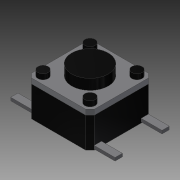
# Autodesk Inventor part: PZ_PushButton
Saved by Autodesk Inventor 2015 (Build 190159000, 159)
## iProperties
Created: 2015-10-19
Part Number: PZ_PushButton
Material: Genérico
Document SubType Name: Modeling
Designer: X1
Density: 1 g/cm^3
Appearance: Valor por defecto
Author: X1
Autodesk Inventor part; units mm, degrees
ref_plane "YZ Plane" through (0, 0, 0) normal (1, 0, 0) x (0, 1, 0)
ref_plane "XZ Plane" through (0, 0, 0) normal (0, 1, 0) x (-1, 0, 0)
sketch "Boceto1" plane through (0, 0, 0) normal (0, 0, 1) x (1, 0, 0)
  line L0 (-7.8, 0) -> (4.8, 0) projected
  line L1 (0, -4.2) -> (0, 4.2) projected
  line L2 (-2.6, 3) -> (2.6, 3)
  line L3 (3, 2.6) -> (3, -2.6)
  line L4 (2.6, -3) -> (-2.6, -3)
  line L5 (-3, -2.6) -> (-3, 2.6)
  circle A0 centre (-2.25, 2.25) radius 0.5
  circle A1 centre (-2.25, -2.25) radius 0.5
  circle A2 centre (2.25, 2.25) radius 0.5
  circle A3 centre (2.25, -2.25) radius 0.5
  circle A4 centre (0, 0) radius 1.75
  line L6 (-2.6, 3) -> (-3, 2.6)
  line L7 (2.6, 3) -> (3, 2.6)
  line L8 (3, -2.6) -> (2.6, -3)
  line L9 (-3, -2.6) -> (-2.6, -3)
  point P0 (-3, 3)
  point P1 (3, -3)
  point P2 (3, 3)
  point P3 (-3, -3)
  dimension "d0" = 6
  dimension "d1" = 6
  dimension "d2" = 4.5
  dimension "d4" = 4.5
  dimension "d5" = 1
  dimension "d6" = 3.5
  dimension "d7" = 0.4
  dimension "d8" = 0.4
  dimension "d9" = 0.4
  dimension "d10" = 0.4
  dimension "d11" = 0.4
  dimension "d12" = 0.4
  dimension "d13" = 0.4
  dimension "d14" = 0.4
  constraints: 16 end point, 8 point on line, 5 centre point, 2 parallel, 1 coincident, 1 horizontal, 1 perpendicular, 5 other
  measures "d0" distance of point (3, -3) point (-3, -3)
  measures "d1" distance of point (3, 3) point (3, -3)
  measures "d2" distance of A0.centre A1.centre
  measures "d4" distance of A2.centre A0.centre
  measures "d5" diameter of A0
  measures "d6" diameter of A4
  measures "d7" distance of L2.start point (-3, 3)
  measures "d8" distance of L5.end point (-3, 3)
  measures "d9" distance of L2.end point (3, 3)
  measures "d10" distance of L3.start point (3, 3)
  measures "d11" distance of L3.end point (3, -3)
  measures "d12" distance of L4.start point (3, -3)
  measures "d13" distance of L5.start point (-3, -3)
  measures "d14" distance of L4.end point (-3, -3)
extrude "Extrusión1" add sketch "Boceto1" against normal blind 3.4 contours L5 L6 L2 L1 A4 L0 | L0 A4 L1 L4 L9 L5 | A4 L1 L0 | L0 L1 A4 | L1 A4 L0 | L0 A4 L1 | L1 L2 L7 L3 L0 A4 | A4 L0 L3 L8 L4 L1 | A0 | A1 | A2 | A3
extrude "Extrusión2" add sketch "Boceto1" along normal blind 0.5 contours A0 | A1 | A2 | A3
extrude "Extrusión3" add sketch "Boceto1" along normal blind 1 contours A4 L1 L0 | L0 L1 A4 | L1 A4 L0 | L0 A4 L1
ref_plane "Plano de trabajo1" through (0, 0, -3) normal (0, 0, 1) x (1, 0, 0)
sketch "Boceto2" plane through (0, 0, -3) normal (0, 0, 1) x (1, 0, 0)
  line L0 (-3, 2.6) -> (-2.6, 3) projected
  line L1 (-2.6, 3) -> (2.6, 3) projected
  line L2 (2.6, 3) -> (3, 2.6) projected
  line L3 (3, 2.6) -> (3, -2.6) projected
  line L4 (3, -2.6) -> (2.6, -3) projected
  line L5 (2.6, -3) -> (-2.6, -3) projected
  line L6 (-2.6, -3) -> (-3, -2.6) projected
  line L7 (-3, -2.6) -> (-3, 2.6) projected
  line L8 (-3, 2.6) -> (-5, 2.6)
  line L9 (-5, 2.6) -> (-5, 1.9)
  line L10 (-5, 1.9) -> (-3, 1.9)
  line L11 (-3, 1.9) -> (-3, 2.6)
  line L12 (-5, 2.25) -> (-3, 2.25)
  line L13 (-7.8, 0) -> (4.8, 0) projected
  line L14 (0, -4.2) -> (0, 4.2) projected
  line L15 (-3, -1.9) -> (-5, -1.9)
  line L16 (-5, -1.9) -> (-5, -2.6)
  line L17 (-5, -2.6) -> (-3, -2.6)
  line L18 (-3, -2.6) -> (-3, -1.9)
  line L19 (5, 2.6) -> (3, 2.6)
  line L20 (3, 2.6) -> (3, 1.9)
  line L21 (3, 1.9) -> (5, 1.9)
  line L22 (5, 1.9) -> (5, 2.6)
  line L23 (5, -1.9) -> (3, -1.9)
  line L24 (3, -1.9) -> (3, -2.6)
  line L25 (3, -2.6) -> (5, -2.6)
  line L26 (5, -2.6) -> (5, -1.9)
  point P0 (0, 0)
  point P1 (-5, -2.25)
  point P2 (-3, -2.25)
  point P3 (3, 2.25)
  point P4 (5, 2.25)
  point P5 (3, -2.25)
  point P6 (5, -2.25)
  dimension "d22" = 2
  dimension "d23" = 0.7
  dimension "d24" = 0.75
  dimension "d27" = 4.5
  dimension "d30" = 8
  constraints: 34 end point, 2 horizontal, 2 midpoint, 2 parallel, 1 perpendicular, 1 point on line, 1 vertical, 30 other
  measures "d22" distance of L10.end L9.end
  measures "d23" distance of L9.end L8.end
  measures "d24" distance between parallel lines of L1 L12
  measures "d27" distance of L9.end L17.start
  measures "d30" distance of L9.end L21.start
extrude "Extrusión4" add sketch "Boceto2" against normal blind 0.3 contours L7 L12 L9 L8 | L7 L10 L9 L12 | L19 L22 L21 L3 | L7 L17 L16 L15 | L23 L26 L25 L3
sketch "Boceto3" plane through (-2.6, 3, 0) normal (0, 1, 0) x (1, 0, 0)
  line L0 (5.2, 0) -> (0, 0) projected
  line L1 (5.2, 0) -> (5.2, 3.4) projected
  line L2 (0, 3.4) -> (5.2, 3.4) projected
  line L3 (0, 0) -> (0, 3.4) projected
  line L4 (5.2, 0.5) -> (0, 0.5)
  line L5 (0, 0) -> (0, 3.4) projected
  point P0 (2.6, 0)
  dimension "d35" = 0.5
  constraints: 2 end point, 2 point on line, 1 perpendicular
  measures "d35" distance between parallel lines of L0 L4
extrude "Extrusión5" add sketch "Boceto3" along normal blind 0.0001 contours L0 L3 L4 L1
mirror "Simetría1" about plane through (0, 0, 0) normal (0, 1, 0) of "Extrusión5"
sketch "Boceto4" plane through (3, -2.6, 0) normal (1, 0, 0) x (0, 0, -1)
  line L0 (3.3, 5.2) -> (3.3, 4.5) projected
  line L1 (3.3, 4.5) -> (3, 4.5) projected
  line L2 (3, 4.5) -> (3, 5.2) projected
  line L3 (0, 5.2) -> (3, 5.2) projected
  line L4 (0, 0) -> (0, 5.2) projected
  line L5 (0, 0) -> (3, 0) projected
  line L6 (3, 0) -> (3, 0.7) projected
  line L7 (3, 0.7) -> (3.3, 0.7) projected
  line L8 (3.3, 0.7) -> (3.3, 0) projected
  line L9 (3.3, 0) -> (3.4, 0) projected
  line L10 (3.4, 5.2) -> (3.4, 0) projected
  line L11 (3.3, 5.2) -> (3.4, 5.2) projected
  line L12 (0.5, 0) -> (0.5, 5.2)
  point P0 (0, 2.6)
  dimension "d38" = 0.5
  constraints: 2 end point, 2 point on line, 1 perpendicular
  measures "d38" distance between parallel lines of L4 L12
extrude "Extrusión6" add sketch "Boceto4" along normal blind 0.0001 contours L12 L5 L4 L3
mirror "Simetría2" about plane through (0, 0, 0) normal (1, 0, 0) of "Extrusión6"
sketch "Boceto5" plane through (3, -2.6, -3) normal (0.7071, -0.7071, 0) x (-0.7071, -0.7071, 0)
  line L0 (0.5657, -2.5) -> (0, -2.5)
  line L1 (0, -2.5) -> (0, -3)
  line L2 (0, -3) -> (0, -2.5) projected
  line L3 (0, -3) -> (0.5657, -3)
  line L4 (0.5657, -3) -> (0, -3) projected
  line L5 (0.5657, -3) -> (0.5657, -2.5)
  line L6 (0.5657, -3) -> (0.5657, -2.5) projected
  point P0 (0.2828, -3)
  constraints: 8 end point, 3 collinear, 1 horizontal
extrude "Extrusión7" add sketch "Boceto5" along normal blind 0.0001
sketch "Boceto6" plane through (3, 2.6, -3.3) normal (0.7071, 0.7071, 0) x (-0.7071, 0.7071, 0)
  line L0 (-0.0001, 3.3) -> (0.5657, 3.3)
  line L1 (0.5657, 3.3) -> (0, 3.3) projected
  line L2 (0.5658, 3.3) -> (0.5658, 2.8) projected
  line L3 (0.5657, 3.3) -> (0.5658, 2.8)
  line L4 (0.5658, 2.8) -> (0, 2.8)
  line L5 (0, 2.8) -> (-0.0001, 3.3)
  point P0 (0.2828, 3.3)
  constraints: 8 end point, 1 collinear
extrude "Extrusión8" add sketch "Boceto6" along normal blind 0.0001
sketch "Boceto7" plane through (-3, -2.6, -3) normal (-0.7071, -0.7071, 0) x (-0.7071, 0.7071, 0)
  line L0 (0, -2.5) -> (-0.5657, -2.5)
  line L1 (-0.5658, -2.5) -> (-0.5658, -3) projected
  line L2 (-0.5657, -2.5) -> (-0.5658, -3)
  line L3 (-0.5658, -3) -> (0, -3)
  line L4 (0, -3) -> (-0.5657, -3) projected
  line L5 (0, -3) -> (0, -2.5)
  point P0 (-0.2828, -3)
  constraints: 8 end point, 1 collinear, 1 horizontal, 1 perpendicular
extrude "Extrusión9" add sketch "Boceto7" along normal blind 0.0001
sketch "Boceto8" plane through (-3, 2.6, -3.3) normal (-0.7071, 0.7071, 0) x (-0.7071, -0.7071, 0)
  line L0 (0, 3.3) -> (-0.5657, 3.3)
  line L1 (-0.5657, 3.3) -> (0, 3.3) projected
  line L2 (-0.5657, 3.3) -> (-0.5657, 2.8)
  line L3 (-0.5657, 2.8) -> (0, 2.8)
  line L4 (-0.5657, 2.8) -> (0, 2.8) projected
  line L5 (0, 2.8) -> (0, 3.3)
  line L6 (0, 3.3) -> (0, 2.8) projected
  point P0 (-0.2828, 3.3)
  constraints: 8 end point, 3 collinear, 1 perpendicular
extrude "Extrusión10" add sketch "Boceto8" along normal blind 0.0001
equation "\"d10\" = d9"
